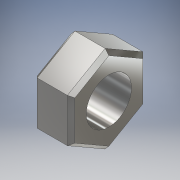
# Autodesk Inventor part: 04-01-Гайка М10
Saved by Autodesk Inventor 2017 SP1 (Build 210196100, 196)
## iProperties
Part Number: 04-01-Гайка М10
Material: Типовые
Document SubType Name: Modeling
Designer: sbnnl
Density: 1 g/cm^3
Appearance: Хром - полированный
Author: sbnnl
Autodesk Inventor part; units mm, degrees
ref_plane "YZ Plane" through (0, 0, 0) normal (1, 0, 0) x (0, 1, 0)
ref_plane "XZ Plane" through (0, 0, 0) normal (0, 1, 0) x (-1, 0, 0)
ref_plane "XY Plane" through (0, 0, 0) normal (0, 0, 1) x (1, 0, 0)
sketch "Эскиз1" plane through (0, 0, 0) normal (1, 0, 0) x (0, 1, 0)
  line L0 (0, -5.7735) -> (-5, -2.8868)
  line L1 (-5, -2.8868) -> (-5, 2.8868)
  line L2 (-5, 2.8868) -> (0, 5.7735)
  line L3 (0, 5.7735) -> (5, 2.8868)
  line L4 (5, 2.8868) -> (5, -2.8868)
  line L5 (5, -2.8868) -> (0, -5.7735)
  circle A0 centre (0, 0) radius 3
  dimension "d0" = 10
  dimension "d1" = 6
  constraints: 12 end point, 2 coincident, 1 centre point, 1 vertical, 13 other
  measures "d0" distance between parallel lines of L1 L4
  measures "d1" diameter of A0
extrude "Выдавливание1" add sketch "Эскиз1" along normal blind 5
chamfer "Фаска1" distance 0.5 angle 45 12 edges at (5, 2.5, 4.3301) (5, 5, 0) (5, 2.5, -4.3301) (5, -2.5, -4.3301) (5, -5, 0) (5, -2.5, 4.3301) (0, 2.5, 4.3301) (0, -2.5, 4.3301) (0, 5, 0) (0, 2.5, -4.3301) (0, -2.5, -4.3301) (0, -5, 0)
